Autodesk Fusion 360 part; units mm, degrees
(part 3 of 3)
  spline S35 degree 5 poles (10.6114, 19.2717) (10.6024, 19.2665) (10.5842, 19.256) (10.557, 19.2403) (10.5209, 19.2193) (10.476, 19.1928) (10.4312, 19.1661) (10.3866, 19.1393) (10.3422, 19.1123) (10.298, 19.0851) (10.254, 19.0578) (10.2102, 19.0302) (10.1666, 19.0026) (10.1231, 18.9747) (10.0799, 18.9466) (10.0369, 18.9184) (9.9941, 18.8901) (9.9515, 18.8615) (9.9091, 18.8328) (9.8669, 18.8038) (9.8249, 18.7748) (9.7832, 18.7455) (9.7416, 18.7161) (9.7003, 18.6865) (9.6592, 18.6567) (9.6183, 18.6267) (9.5776, 18.5966) (9.5372, 18.5662) (9.497, 18.5357) (9.457, 18.5051) (9.4173, 18.4742) (9.3778, 18.4432) (9.3385, 18.412) (9.2995, 18.3806) (9.2607, 18.349) (9.2222, 18.3172) (9.1839, 18.2853) (9.1459, 18.2531) (9.1082, 18.2208) (9.0707, 18.1883) (9.0335, 18.1556) (8.9965, 18.1227) (8.9598, 18.0896) (8.9234, 18.0564) (8.8873, 18.0229) (8.8515, 17.9892) (8.816, 17.9554) (8.7808, 17.9213) (8.7458, 17.8871) (8.7112, 17.8526) (8.6769, 17.8179) (8.643, 17.7831) (8.6093, 17.748) (8.576, 17.7127) (8.5431, 17.6772) (8.5105, 17.6415) (8.4782, 17.6055) (8.4464, 17.5693) (8.415, 17.5329) (8.384, 17.4962) (8.3534, 17.4593) (8.3232, 17.4221) (8.2934, 17.3847) (8.264, 17.3471) (8.2352, 17.3092) (8.2069, 17.2709) (8.1792, 17.2323) (8.1523, 17.1934) (8.1261, 17.154) (8.1007, 17.1142) (8.0762, 17.074) (8.0573, 17.0414) (8.0434, 17.0168) (8.0344, 17.0003) (8.0299, 16.992) knots -1 -1 -1 -1 -1 -1 -0.98571429 -0.97142857 -0.95714286 -0.94285714 -0.92857143 -0.91428571 -0.9 -0.88571429 -0.87142857 -0.85714286 -0.84285714 -0.82857143 -0.81428571 -0.8 -0.78571429 -0.77142857 -0.75714286 -0.74285714 -0.72857143 -0.71428571 -0.7 -0.68571429 -0.67142857 -0.65714286 -0.64285714 -0.62857143 -0.61428571 -0.6 -0.58571429 -0.57142857 -0.55714286 -0.54285714 -0.52857143 -0.51428571 -0.5 -0.48571429 -0.47142857 -0.45714286 -0.44285714 -0.42857143 -0.41428571 -0.4 -0.38571429 -0.37142857 -0.35714286 -0.34285714 -0.32857143 -0.31428571 -0.3 -0.28571429 -0.27142857 -0.25714286 -0.24285714 -0.22857143 -0.21428571 -0.2 -0.18571429 -0.17142857 -0.15714286 -0.14285714 -0.12857143 -0.11428571 -0.1 -0.08571429 -0.07142857 -0.05714286 -0.04285714 -0.02857143 -0.01428571 0 0 0 0 0 0
  line L71 (8.0299, 16.992) -> (7.6878, 16.268)
  arc A53 (7.0347, 16.0238) -> (7.6878, 16.268) centre (7.2357, 16.4816) ccw
  arc A54 (7.0347, 16.0238) -> (5.868, 16.4869) centre (0, 0) ccw
  arc A55 (5.5602, 17.1124) -> (5.868, 16.4869) centre (6.0357, 16.9579) ccw
  line L72 (5.5602, 17.1124) -> (5.8076, 17.874)
  spline S36 degree 5 poles (5.8076, 17.874) (5.81, 17.8831) (5.8148, 17.9013) (5.8216, 17.9287) (5.8301, 17.9654) (5.8399, 18.0115) (5.8487, 18.0579) (5.8566, 18.1045) (5.8637, 18.1513) (5.8701, 18.1983) (5.8757, 18.2456) (5.8807, 18.293) (5.8852, 18.3405) (5.8891, 18.3882) (5.8926, 18.4359) (5.8957, 18.4838) (5.8982, 18.5317) (5.9003, 18.5798) (5.902, 18.628) (5.9032, 18.6762) (5.904, 18.7246) (5.9043, 18.773) (5.9043, 18.8216) (5.9039, 18.8702) (5.903, 18.9188) (5.9019, 18.9676) (5.9003, 19.0164) (5.8984, 19.0653) (5.8961, 19.1142) (5.8935, 19.1632) (5.8905, 19.2123) (5.8871, 19.2614) (5.8835, 19.3106) (5.8794, 19.3598) (5.8751, 19.4091) (5.8704, 19.4584) (5.8654, 19.5078) (5.8601, 19.5572) (5.8545, 19.6066) (5.8486, 19.6561) (5.8423, 19.7057) (5.8357, 19.7552) (5.8289, 19.8048) (5.8217, 19.8545) (5.8142, 19.9042) (5.8065, 19.9539) (5.7984, 20.0036) (5.7901, 20.0534) (5.7814, 20.1032) (5.7725, 20.153) (5.7633, 20.2029) (5.7538, 20.2527) (5.744, 20.3026) (5.734, 20.3525) (5.7236, 20.4025) (5.713, 20.4524) (5.7021, 20.5024) (5.691, 20.5524) (5.6796, 20.6024) (5.6679, 20.6524) (5.6559, 20.7024) (5.6437, 20.7525) (5.6312, 20.8026) (5.6184, 20.8526) (5.6054, 20.9027) (5.5921, 20.9528) (5.5786, 21.0029) (5.5648, 21.053) (5.5507, 21.1031) (5.5364, 21.1532) (5.5219, 21.2033) (5.51, 21.2434) (5.501, 21.2734) (5.4949, 21.2935) (5.4919, 21.3035) knots 0 0 0 0 0 0 0.01428571 0.02857143 0.04285714 0.05714286 0.07142857 0.08571429 0.1 0.11428571 0.12857143 0.14285714 0.15714286 0.17142857 0.18571429 0.2 0.21428571 0.22857143 0.24285714 0.25714286 0.27142857 0.28571429 0.3 0.31428571 0.32857143 0.34285714 0.35714286 0.37142857 0.38571429 0.4 0.41428571 0.42857143 0.44285714 0.45714286 0.47142857 0.48571429 0.5 0.51428571 0.52857143 0.54285714 0.55714286 0.57142857 0.58571429 0.6 0.61428571 0.62857143 0.64285714 0.65714286 0.67142857 0.68571429 0.7 0.71428571 0.72857143 0.74285714 0.75714286 0.77142857 0.78571429 0.8 0.81428571 0.82857143 0.84285714 0.85714286 0.87142857 0.88571429 0.9 0.91428571 0.92857143 0.94285714 0.95714286 0.97142857 0.98571429 1 1 1 1 1 1
  line L73 (5.4919, 21.3035) -> (4.8168, 21.4662)
  line L74 (4.8168, 21.4662) -> (4.1368, 21.6076)
  spline S37 degree 5 poles (4.1368, 21.6076) (4.1298, 21.5998) (4.1157, 21.5843) (4.0948, 21.5609) (4.0669, 21.5297) (4.0323, 21.4907) (3.998, 21.4515) (3.9639, 21.4122) (3.93, 21.3728) (3.8964, 21.3333) (3.863, 21.2937) (3.8298, 21.254) (3.7969, 21.2141) (3.7642, 21.1742) (3.7317, 21.1342) (3.6996, 21.0941) (3.6676, 21.0539) (3.6359, 21.0135) (3.6045, 20.9731) (3.5733, 20.9326) (3.5423, 20.8919) (3.5117, 20.8512) (3.4812, 20.8104) (3.4511, 20.7694) (3.4212, 20.7284) (3.3916, 20.6873) (3.3622, 20.646) (3.3331, 20.6047) (3.3043, 20.5633) (3.2758, 20.5217) (3.2475, 20.4801) (3.2195, 20.4384) (3.1918, 20.3966) (3.1644, 20.3546) (3.1373, 20.3126) (3.1105, 20.2705) (3.084, 20.2283) (3.0578, 20.186) (3.0318, 20.1436) (3.0062, 20.1011) (2.9809, 20.0585) (2.956, 20.0158) (2.9313, 19.973) (2.907, 19.9301) (2.883, 19.8871) (2.8593, 19.844) (2.836, 19.8009) (2.813, 19.7576) (2.7904, 19.7142) (2.7681, 19.6708) (2.7462, 19.6272) (2.7247, 19.5835) (2.7035, 19.5398) (2.6828, 19.4959) (2.6624, 19.452) (2.6424, 19.4079) (2.6229, 19.3638) (2.6038, 19.3195) (2.5852, 19.2751) (2.567, 19.2307) (2.5493, 19.1861) (2.5321, 19.1414) (2.5153, 19.0967) (2.499, 19.0518) (2.4833, 19.0068) (2.4682, 18.9617) (2.4538, 18.9164) (2.4402, 18.8711) (2.4275, 18.8255) (2.4157, 18.7798) (2.4048, 18.734) (2.3968, 18.6972) (2.3913, 18.6695) (2.3878, 18.651) (2.3861, 18.6418) knots -1 -1 -1 -1 -1 -1 -0.98571429 -0.97142857 -0.95714286 -0.94285714 -0.92857143 -0.91428571 -0.9 -0.88571429 -0.87142857 -0.85714286 -0.84285714 -0.82857143 -0.81428571 -0.8 -0.78571429 -0.77142857 -0.75714286 -0.74285714 -0.72857143 -0.71428571 -0.7 -0.68571429 -0.67142857 -0.65714286 -0.64285714 -0.62857143 -0.61428571 -0.6 -0.58571429 -0.57142857 -0.55714286 -0.54285714 -0.52857143 -0.51428571 -0.5 -0.48571429 -0.47142857 -0.45714286 -0.44285714 -0.42857143 -0.41428571 -0.4 -0.38571429 -0.37142857 -0.35714286 -0.34285714 -0.32857143 -0.31428571 -0.3 -0.28571429 -0.27142857 -0.25714286 -0.24285714 -0.22857143 -0.21428571 -0.2 -0.18571429 -0.17142857 -0.15714286 -0.14285714 -0.12857143 -0.11428571 -0.1 -0.08571429 -0.07142857 -0.05714286 -0.04285714 -0.02857143 -0.01428571 0 0 0 0 0 0
  line L75 (2.3861, 18.6418) -> (2.2844, 17.8474)
  arc A56 (1.7388, 17.4134) -> (2.2844, 17.8474) centre (1.7885, 17.9109) ccw
  arc A57 (1.7388, 17.4134) -> (0.4861, 17.4932) centre (0, 0) ccw
  arc A58 (0, 17.9931) -> (0.4861, 17.4932) centre (0.5, 17.9931) ccw
  line L76 (0, 17.9931) -> (0, 18.7939)
  spline S38 degree 5 poles (0, 18.7939) (-0.0005, 18.8032) (-0.0016, 18.822) (-0.0036, 18.8502) (-0.0068, 18.8877) (-0.0118, 18.9346) (-0.0178, 18.9814) (-0.0246, 19.0282) (-0.0323, 19.0749) (-0.0408, 19.1216) (-0.0501, 19.1683) (-0.06, 19.2149) (-0.0704, 19.2615) (-0.0814, 19.308) (-0.0928, 19.3545) (-0.1047, 19.401) (-0.1171, 19.4474) (-0.1299, 19.4937) (-0.1432, 19.5401) (-0.157, 19.5863) (-0.1712, 19.6326) (-0.1858, 19.6788) (-0.2009, 19.7249) (-0.2163, 19.771) (-0.2321, 19.817) (-0.2483, 19.863) (-0.2649, 19.909) (-0.2818, 19.9549) (-0.2991, 20.0007) (-0.3167, 20.0465) (-0.3347, 20.0922) (-0.3531, 20.1379) (-0.3718, 20.1835) (-0.3908, 20.2291) (-0.4102, 20.2746) (-0.4299, 20.3201) (-0.4499, 20.3655) (-0.4702, 20.4109) (-0.4908, 20.4561) (-0.5118, 20.5014) (-0.533, 20.5466) (-0.5546, 20.5917) (-0.5764, 20.6367) (-0.5986, 20.6817) (-0.6211, 20.7267) (-0.6438, 20.7716) (-0.6668, 20.8164) (-0.6902, 20.8611) (-0.7138, 20.9058) (-0.7376, 20.9504) (-0.7618, 20.995) (-0.7863, 21.0395) (-0.811, 21.0839) (-0.836, 21.1283) (-0.8612, 21.1726) (-0.8867, 21.2168) (-0.9125, 21.261) (-0.9386, 21.3051) (-0.9649, 21.3491) (-0.9915, 21.3931) (-1.0183, 21.437) (-1.0454, 21.4808) (-1.0728, 21.5245) (-1.1004, 21.5682) (-1.1282, 21.6118) (-1.1563, 21.6553) (-1.1847, 21.6988) (-1.2133, 21.7422) (-1.2421, 21.7855) (-1.2712, 21.8287) (-1.3006, 21.8719) (-1.3242, 21.9063) (-1.3421, 21.9321) (-1.354, 21.9493) (-1.36, 21.9579) knots 0 0 0 0 0 0 0.01428571 0.02857143 0.04285714 0.05714286 0.07142857 0.08571429 0.1 0.11428571 0.12857143 0.14285714 0.15714286 0.17142857 0.18571429 0.2 0.21428571 0.22857143 0.24285714 0.25714286 0.27142857 0.28571429 0.3 0.31428571 0.32857143 0.34285714 0.35714286 0.37142857 0.38571429 0.4 0.41428571 0.42857143 0.44285714 0.45714286 0.47142857 0.48571429 0.5 0.51428571 0.52857143 0.54285714 0.55714286 0.57142857 0.58571429 0.6 0.61428571 0.62857143 0.64285714 0.65714286 0.67142857 0.68571429 0.7 0.71428571 0.72857143 0.74285714 0.75714286 0.77142857 0.78571429 0.8 0.81428571 0.82857143 0.84285714 0.85714286 0.87142857 0.88571429 0.9 0.91428571 0.92857143 0.94285714 0.95714286 0.97142857 0.98571429 1 1 1 1 1 1
  line L77 (-1.36, 21.9579) -> (-2.0524, 21.9041)
  line L78 (-2.0524, 21.9041) -> (-2.7428, 21.8284)
  spline S39 degree 5 poles (-2.7428, 21.8284) (-2.747, 21.8188) (-2.7556, 21.7997) (-2.7683, 21.771) (-2.7852, 21.7327) (-2.806, 21.6849) (-2.8265, 21.637) (-2.8468, 21.5891) (-2.8669, 21.5412) (-2.8867, 21.4932) (-2.9062, 21.4452) (-2.9255, 21.3972) (-2.9445, 21.3491) (-2.9632, 21.3011) (-2.9817, 21.253) (-2.9999, 21.2049) (-3.0179, 21.1568) (-3.0356, 21.1086) (-3.053, 21.0604) (-3.0701, 21.0123) (-3.087, 20.964) (-3.1036, 20.9158) (-3.1199, 20.8676) (-3.1359, 20.8193) (-3.1517, 20.7711) (-3.1672, 20.7228) (-3.1823, 20.6745) (-3.1972, 20.6262) (-3.2118, 20.5779) (-3.2261, 20.5296) (-3.2401, 20.4813) (-3.2539, 20.4329) (-3.2673, 20.3846) (-3.2804, 20.3363) (-3.2932, 20.2879) (-3.3057, 20.2396) (-3.3179, 20.1913) (-3.3297, 20.1429) (-3.3413, 20.0946) (-3.3525, 20.0462) (-3.3634, 19.9979) (-3.3739, 19.9496) (-3.3842, 19.9013) (-3.3941, 19.853) (-3.4036, 19.8047) (-3.4128, 19.7564) (-3.4216, 19.7081) (-3.4301, 19.6599) (-3.4382, 19.6116) (-3.446, 19.5634) (-3.4533, 19.5152) (-3.4603, 19.467) (-3.4669, 19.4189) (-3.4731, 19.3707) (-3.4789, 19.3226) (-3.4843, 19.2746) (-3.4892, 19.2265) (-3.4937, 19.1786) (-3.4977, 19.1306) (-3.5012, 19.0827) (-3.5043, 19.0349) (-3.5069, 18.987) (-3.509, 18.9393) (-3.5106, 18.8916) (-3.5117, 18.8439) (-3.5121, 18.7963) (-3.5118, 18.7489) (-3.5107, 18.7015) (-3.5087, 18.6543) (-3.5058, 18.6072) (-3.502, 18.5602) (-3.4982, 18.5227) (-3.4949, 18.4947) (-3.4926, 18.476) (-3.4913, 18.4667) knots -1 -1 -1 -1 -1 -1 -0.98571429 -0.97142857 -0.95714286 -0.94285714 -0.92857143 -0.91428571 -0.9 -0.88571429 -0.87142857 -0.85714286 -0.84285714 -0.82857143 -0.81428571 -0.8 -0.78571429 -0.77142857 -0.75714286 -0.74285714 -0.72857143 -0.71428571 -0.7 -0.68571429 -0.67142857 -0.65714286 -0.64285714 -0.62857143 -0.61428571 -0.6 -0.58571429 -0.57142857 -0.55714286 -0.54285714 -0.52857143 -0.51428571 -0.5 -0.48571429 -0.47142857 -0.45714286 -0.44285714 -0.42857143 -0.41428571 -0.4 -0.38571429 -0.37142857 -0.35714286 -0.34285714 -0.32857143 -0.31428571 -0.3 -0.28571429 -0.27142857 -0.25714286 -0.24285714 -0.22857143 -0.21428571 -0.2 -0.18571429 -0.17142857 -0.15714286 -0.14285714 -0.12857143 -0.11428571 -0.1 -0.08571429 -0.07142857 -0.05714286 -0.04285714 -0.02857143 -0.01428571 0 0 0 0 0 0
  line L79 (-3.4913, 18.4667) -> (-3.3426, 17.6799)
  arc A59 (-3.7274, 17.0984) -> (-3.3426, 17.6799) centre (-3.8339, 17.587) ccw
  arc A60 (-3.7274, 17.0984) -> (-4.9434, 16.7873) centre (0, 0) ccw
  arc A61 (-17.151, -5.4413) -> (-16.9072, -4.9787) centre (-17.2669, -5.0846) ccw
  arc A62 (-17.2206, -3.754) -> (-16.9072, -4.9787) centre (0, 0) ccw
  arc A63 (-17.2206, -3.754) -> (-17.6566, -3.4654) centre (-17.587, -3.8339) ccw
  line L80 (-18.4469, -3.6148) -> (-17.6566, -3.4654)
  spline S40 degree 3 poles (-21.9448, -2.8275) (-21.9231, -2.8373) (-21.9013, -2.847) (-21.8795, -2.8568) (-21.1038, -3.2048) (-20.3139, -3.4618) (-19.5249, -3.5782) (-19.1675, -3.6309) (-18.8078, -3.6627) (-18.4503, -3.6152) (-18.4491, -3.6151) (-18.448, -3.6149) (-18.4469, -3.6148) knots -1.019521 -1.019521 -1.019521 -1.019521 -1 -1 -1 -0.311758 -0.311758 -0.311758 0 0 0 0.001043 0.001043 0.001043 0.001043
  line L81 (-22.0285, -2.0641) -> (-21.9448, -2.8275)
  line L82 (-22.0881, -1.2984) -> (-22.0285, -2.0641)
  spline S41 degree 3 poles (-18.7973, 0.125) (-18.7984, 0.1249) (-18.7996, 0.1249) (-18.8007, 0.1248) (-19.3678, 0.0936) (-19.9052, -0.1072) (-20.433, -0.3432) (-20.9804, -0.5879) (-21.5134, -0.8979) (-22.0294, -1.2575) (-22.049, -1.2711) (-22.0685, -1.2847) (-22.0881, -1.2984) knots -0.001043 -0.001043 -0.001043 -0.001043 0 0 0 0.490911 0.490911 0.490911 1 1 1 1.019521 1.019521 1.019521 1.019521
  line L83 (-17.9931, 0.125) -> (-18.7973, 0.125)
  arc A64 (-17.9931, 0.125) -> (-17.6182, 0.4896) centre (-17.9931, 0.5) ccw
  arc A65 (-17.5378, 1.7512) -> (-17.6182, 0.4896) centre (0, 0) ccw
  arc A66 (-17.5378, 1.7512) -> (-17.8633, 2.1604) centre (-17.9109, 1.7885) ccw
  line L84 (-18.661, 2.2625) -> (-17.8633, 2.1604)
  spline S42 degree 3 poles (-21.7445, 4.0922) (-21.7268, 4.0762) (-21.7091, 4.0602) (-21.6915, 4.0442) (-21.0612, 3.4735) (-20.3894, 2.985) (-19.675, 2.6305) (-19.3514, 2.4699) (-19.0191, 2.3285) (-18.6644, 2.2632) (-18.6633, 2.2629) (-18.6622, 2.2627) (-18.661, 2.2625) knots -1.019521 -1.019521 -1.019521 -1.019521 -1 -1 -1 -0.311758 -0.311758 -0.311758 0 0 0 0.001043 0.001043 0.001043 0.001043
  line L85 (-21.5882, 4.8441) -> (-21.7445, 4.0922)
  line L86 (-21.4082, 5.5908) -> (-21.5882, 4.8441)
  spline S43 degree 3 poles (-17.8387, 5.9276) (-17.8398, 5.9279) (-17.8409, 5.9281) (-17.842, 5.9284) (-18.391, 6.074) (-18.9641, 6.0491) (-19.539, 5.9878) (-20.1352, 5.9242) (-20.7379, 5.794) (-21.3398, 5.6115) (-21.3626, 5.6046) (-21.3854, 5.5977) (-21.4082, 5.5908) knots -0.001043 -0.001043 -0.001043 -0.001043 0 0 0 0.490911 0.490911 0.490911 1 1 1 1.019521 1.019521 1.019521 1.019521
  line L87 (-17.0738, 5.679) -> (-17.8387, 5.9276)
  arc A67 (-17.0738, 5.679) -> (-16.6046, 5.9099) centre (-16.9579, 6.0357) ccw
  arc A68 (-16.1383, 7.085) -> (-16.6046, 5.9099) centre (0, 0) ccw
  arc A69 (-16.1383, 7.085) -> (-16.3214, 7.5748) centre (-16.4816, 7.2357) ccw
  line L88 (-17.0485, 7.9184) -> (-16.3214, 7.5748)
  spline S44 degree 3 poles (-19.4157, 10.6113) (-19.4038, 10.5906) (-19.392, 10.5699) (-19.3801, 10.5493) (-18.9571, 9.8117) (-18.4691, 9.1396) (-17.8992, 8.5817) (-17.641, 8.329) (-17.3687, 8.0918) (-17.0516, 7.92) (-17.0506, 7.9195) (-17.0496, 7.9189) (-17.0485, 7.9184) knots -1.019521 -1.019521 -1.019521 -1.019521 -1 -1 -1 -0.311758 -0.311758 -0.311758 0 0 0 0.001043 0.001043 0.001043 0.001043
  line L89 (-19.0347, 11.2782) -> (-19.4157, 10.6113)
  line L90 (-18.6328, 11.9326) -> (-19.0347, 11.2782)
  spline S45 degree 3 poles (-15.1339, 11.1499) (-15.1348, 11.1505) (-15.1358, 11.1511) (-15.1367, 11.1518) (-15.6139, 11.4599) (-16.1667, 11.6132) (-16.7324, 11.7326) (-17.319, 11.8564) (-17.9325, 11.9188) (-18.5613, 11.9312) (-18.5851, 11.9317) (-18.609, 11.9322) (-18.6328, 11.9326) knots -0.001043 -0.001043 -0.001043 -0.001043 0 0 0 0.490911 0.490911 0.490911 1 1 1 1.019521 1.019521 1.019521 1.019521
  line L91 (-14.4832, 10.6772) -> (-15.1339, 11.1499)
  arc A70 (-14.4832, 10.6772) -> (-13.9657, 10.7518) centre (-14.2628, 10.9806) ccw
  arc A71 (-13.159, 11.7252) -> (-13.9657, 10.7518) centre (0, 0) ccw
  arc A72 (-13.159, 11.7252) -> (-13.1819, 12.2476) centre (-13.439, 11.9747) ccw
  line L92 (-13.7672, 12.7991) -> (-13.1819, 12.2476)
  spline S46 degree 3 poles (-15.1864, 16.0918) (-15.1815, 16.0684) (-15.1766, 16.0451) (-15.1717, 16.0217) (-14.9972, 15.1896) (-14.7409, 14.3995) (-14.3712, 13.6928) (-14.2038, 13.3727) (-14.0181, 13.063) (-13.7696, 12.8016) (-13.7688, 12.8008) (-13.768, 12.7999) (-13.7672, 12.7991) knots -1.019521 -1.019521 -1.019521 -1.019521 -1 -1 -1 -0.311758 -0.311758 -0.311758 0 0 0 0.001043 0.001043 0.001043 0.001043
  line L93 (-14.6179, 16.6082) -> (-15.1864, 16.0918)
  line L94 (-14.0335, 17.1065) -> (-14.6179, 16.6082)
  spline S47 degree 3 poles (-10.9476, 15.2808) (-10.9484, 15.2817) (-10.9491, 15.2826) (-10.9498, 15.2835) (-11.3084, 15.7239) (-11.7867, 16.0406) (-12.2879, 16.3289) (-12.8075, 16.6279) (-13.3717, 16.8769) (-13.9659, 17.083) (-13.9884, 17.0908) (-14.0109, 17.0987) (-14.0335, 17.1065) knots -0.001043 -0.001043 -0.001043 -0.001043 0 0 0 0.490911 0.490911 0.490911 1 1 1 1.019521 1.019521 1.019521 1.019521
  line L95 (-10.4749, 14.6302) -> (-10.9476, 15.2808)
  arc A73 (-10.4749, 14.6302) -> (-9.9596, 14.5412) centre (-10.1715, 14.8506) ccw
  arc A74 (-8.8917, 15.2177) -> (-9.9596, 14.5412) centre (0, 0) ccw
  arc A75 (-8.8917, 15.2177) -> (-8.752, 15.7216) centre (-9.0809, 15.5415) ccw
  line L96 (-9.1383, 16.427) -> (-8.752, 15.7216)
  spline S48 degree 3 poles (-9.4705, 19.997) (-9.473, 19.9733) (-9.4756, 19.9496) (-9.4781, 19.9259) (-9.5694, 19.0805) (-9.5697, 18.2499) (-9.4366, 17.4636) (-9.3763, 17.1074) (-9.2954, 16.7555) (-9.1397, 16.4301) (-9.1392, 16.429) (-9.1388, 16.428) (-9.1383, 16.427) knots -1.019521 -1.019521 -1.019521 -1.019521 -1 -1 -1 -0.311758 -0.311758 -0.311758 0 0 0 0.001043 0.001043 0.001043 0.001043
  line L97 (-8.7702, 20.3125) -> (-9.4705, 19.997)
  line L98 (-8.0604, 20.6058) -> (-8.7702, 20.3125)
  spline S49 degree 3 poles (-5.6898, 17.9159) (-5.6902, 17.917) (-5.6906, 17.918) (-5.691, 17.9191) (-5.8959, 18.4488) (-6.253, 18.8978) (-6.6405, 19.3269) (-7.0424, 19.7718) (-7.502, 20.183) (-8.0034, 20.5626) (-8.0224, 20.577) (-8.0414, 20.5914) (-8.0604, 20.6058) knots -0.001043 -0.001043 -0.001043 -0.001043 0 0 0 0.490911 0.490911 0.490911 1 1 1 1.019521 1.019521 1.019521 1.019521
  line L99 (-5.4413, 17.151) -> (-5.6898, 17.9159)
  arc A76 (-5.4413, 17.151) -> (-4.9787, 16.9072) centre (-5.0846, 17.2669) ccw
  arc A77 (-3.754, 17.2206) -> (-4.9787, 16.9072) centre (0, 0) ccw
  arc A78 (-3.754, 17.2206) -> (-3.4654, 17.6566) centre (-3.8339, 17.587) ccw
  line L100 (-3.6148, 18.4469) -> (-3.4654, 17.6566)
  spline S50 degree 3 poles (-2.8275, 21.9448) (-2.8373, 21.9231) (-2.847, 21.9013) (-2.8568, 21.8795) (-3.2048, 21.1038) (-3.4618, 20.3139) (-3.5782, 19.5249) (-3.6309, 19.1675) (-3.6627, 18.8078) (-3.6152, 18.4503) (-3.6151, 18.4491) (-3.6149, 18.448) (-3.6148, 18.4469) knots -1.019521 -1.019521 -1.019521 -1.019521 -1 -1 -1 -0.311758 -0.311758 -0.311758 0 0 0 0.001043 0.001043 0.001043 0.001043
  line L101 (-2.0641, 22.0285) -> (-2.8275, 21.9448)
  line L102 (-1.2984, 22.0881) -> (-2.0641, 22.0285)
  spline S51 degree 3 poles (0.125, 18.7973) (0.1249, 18.7984) (0.1249, 18.7996) (0.1248, 18.8007) (0.0936, 19.3678) (-0.1072, 19.9052) (-0.3432, 20.433) (-0.5879, 20.9804) (-0.8979, 21.5134) (-1.2575, 22.0294) (-1.2711, 22.049) (-1.2847, 22.0685) (-1.2984, 22.0881) knots -0.001043 -0.001043 -0.001043 -0.001043 0 0 0 0.490911 0.490911 0.490911 1 1 1 1.019521 1.019521 1.019521 1.019521
  line L103 (0.125, 17.9931) -> (0.125, 18.7973)
  arc A79 (0.125, 17.9931) -> (0.4896, 17.6182) centre (0.5, 17.9931) ccw
  arc A80 (1.7512, 17.5378) -> (0.4896, 17.6182) centre (0, 0) ccw
  arc A81 (1.7512, 17.5378) -> (2.1604, 17.8633) centre (1.7885, 17.9109) ccw
  line L104 (2.2625, 18.661) -> (2.1604, 17.8633)
  spline S52 degree 3 poles (4.0922, 21.7445) (4.0762, 21.7268) (4.0602, 21.7091) (4.0442, 21.6915) (3.4735, 21.0612) (2.985, 20.3894) (2.6305, 19.675) (2.4699, 19.3514) (2.3285, 19.0191) (2.2632, 18.6644) (2.2629, 18.6633) (2.2627, 18.6622) (2.2625, 18.661) knots -1.019521 -1.019521 -1.019521 -1.019521 -1 -1 -1 -0.311758 -0.311758 -0.311758 0 0 0 0.001043 0.001043 0.001043 0.001043
  line L105 (4.8441, 21.5882) -> (4.0922, 21.7445)
  line L106 (5.5908, 21.4082) -> (4.8441, 21.5882)
  spline S53 degree 3 poles (5.9276, 17.8387) (5.9279, 17.8398) (5.9281, 17.8409) (5.9284, 17.842) (6.074, 18.391) (6.0491, 18.9641) (5.9878, 19.539) (5.9242, 20.1352) (5.794, 20.7379) (5.6115, 21.3398) (5.6046, 21.3626) (5.5977, 21.3854) (5.5908, 21.4082) knots -0.001043 -0.001043 -0.001043 -0.001043 0 0 0 0.490911 0.490911 0.490911 1 1 1 1.019521 1.019521 1.019521 1.019521
  line L107 (5.679, 17.0738) -> (5.9276, 17.8387)
  arc A82 (5.679, 17.0738) -> (5.9099, 16.6046) centre (6.0357, 16.9579) ccw
  arc A83 (7.085, 16.1383) -> (5.9099, 16.6046) centre (0, 0) ccw
  arc A84 (7.085, 16.1383) -> (7.5748, 16.3214) centre (7.2357, 16.4816) ccw
  line L108 (7.9184, 17.0485) -> (7.5748, 16.3214)
  spline S54 degree 3 poles (10.6113, 19.4157) (10.5906, 19.4038) (10.5699, 19.392) (10.5493, 19.3801) (9.8117, 18.9571) (9.1396, 18.4691) (8.5817, 17.8992) (8.329, 17.641) (8.0918, 17.3687) (7.92, 17.0516) (7.9195, 17.0506) (7.9189, 17.0496) (7.9184, 17.0485) knots -1.019521 -1.019521 -1.019521 -1.019521 -1 -1 -1 -0.311758 -0.311758 -0.311758 0 0 0 0.001043 0.001043 0.001043 0.001043
  line L109 (11.2782, 19.0347) -> (10.6113, 19.4157)
  line L110 (11.9326, 18.6328) -> (11.2782, 19.0347)
  spline S55 degree 3 poles (11.1499, 15.1339) (11.1505, 15.1348) (11.1511, 15.1358) (11.1518, 15.1367) (11.4599, 15.6139) (11.6132, 16.1667) (11.7326, 16.7324) (11.8564, 17.319) (11.9188, 17.9325) (11.9312, 18.5613) (11.9317, 18.5851) (11.9322, 18.609) (11.9326, 18.6328) knots -0.001043 -0.001043 -0.001043 -0.001043 0 0 0 0.490911 0.490911 0.490911 1 1 1 1.019521 1.019521 1.019521 1.019521
  line L111 (10.6772, 14.4832) -> (11.1499, 15.1339)
  arc A85 (10.6772, 14.4832) -> (10.7518, 13.9657) centre (10.9806, 14.2628) ccw
  arc A86 (11.7252, 13.159) -> (10.7518, 13.9657) centre (0, 0) ccw
  arc A87 (11.7252, 13.159) -> (12.2476, 13.1819) centre (11.9747, 13.439) ccw
  line L112 (12.7991, 13.7672) -> (12.2476, 13.1819)
  spline S56 degree 3 poles (16.0918, 15.1864) (16.0684, 15.1815) (16.0451, 15.1766) (16.0217, 15.1717) (15.1896, 14.9972) (14.3995, 14.7409) (13.6928, 14.3712) (13.3727, 14.2038) (13.063, 14.0181) (12.8016, 13.7696) (12.8008, 13.7688) (12.7999, 13.768) (12.7991, 13.7672) knots -1.019521 -1.019521 -1.019521 -1.019521 -1 -1 -1 -0.311758 -0.311758 -0.311758 0 0 0 0.001043 0.001043 0.001043 0.001043
  line L113 (16.6082, 14.6179) -> (16.0918, 15.1864)
  line L114 (17.1065, 14.0335) -> (16.6082, 14.6179)
  spline S57 degree 3 poles (15.2808, 10.9476) (15.2817, 10.9484) (15.2826, 10.9491) (15.2835, 10.9498) (15.7239, 11.3084) (16.0406, 11.7867) (16.3289, 12.2879) (16.6279, 12.8075) (16.8769, 13.3717) (17.083, 13.9659) (17.0908, 13.9884) (17.0987, 14.0109) (17.1065, 14.0335) knots -0.001043 -0.001043 -0.001043 -0.001043 0 0 0 0.490911 0.490911 0.490911 1 1 1 1.019521 1.019521 1.019521 1.019521
  line L115 (14.6302, 10.4749) -> (15.2808, 10.9476)
  arc A88 (14.6302, 10.4749) -> (14.5412, 9.9596) centre (14.8506, 10.1715) ccw
  arc A89 (15.2177, 8.8917) -> (14.5412, 9.9596) centre (0, 0) ccw
  arc A90 (15.2177, 8.8917) -> (15.7216, 8.752) centre (15.5415, 9.0809) ccw
  line L116 (16.427, 9.1383) -> (15.7216, 8.752)
  spline S58 degree 3 poles (19.997, 9.4705) (19.9733, 9.473) (19.9496, 9.4756) (19.9259, 9.4781) (19.0805, 9.5694) (18.2499, 9.5697) (17.4636, 9.4366) (17.1074, 9.3763) (16.7555, 9.2954) (16.4301, 9.1397) (16.429, 9.1392) (16.428, 9.1388) (16.427, 9.1383) knots -1.019521 -1.019521 -1.019521 -1.019521 -1 -1 -1 -0.311758 -0.311758 -0.311758 0 0 0 0.001043 0.001043 0.001043 0.001043
  line L117 (20.3125, 8.7702) -> (19.997, 9.4705)
  line L118 (20.6058, 8.0604) -> (20.3125, 8.7702)
  spline S59 degree 3 poles (17.9159, 5.6898) (17.917, 5.6902) (17.918, 5.6906) (17.9191, 5.691) (18.4488, 5.8959) (18.8978, 6.253) (19.3269, 6.6405) (19.7718, 7.0424) (20.183, 7.502) (20.5626, 8.0034) (20.577, 8.0224) (20.5914, 8.0414) (20.6058, 8.0604) knots -0.001043 -0.001043 -0.001043 -0.001043 0 0 0 0.490911 0.490911 0.490911 1 1 1 1.019521 1.019521 1.019521 1.019521
  line L119 (17.151, 5.4413) -> (17.9159, 5.6898)
  arc A91 (17.151, 5.4413) -> (16.9072, 4.9787) centre (17.2669, 5.0846) ccw
  arc A92 (17.2206, 3.754) -> (16.9072, 4.9787) centre (0, 0) ccw
  arc A93 (17.2206, 3.754) -> (17.6566, 3.4654) centre (17.587, 3.8339) ccw
  line L120 (18.4469, 3.6148) -> (17.6566, 3.4654)
  spline S60 degree 3 poles (21.9448, 2.8275) (21.9231, 2.8373) (21.9013, 2.847) (21.8795, 2.8568) (21.1038, 3.2048) (20.3139, 3.4618) (19.5249, 3.5782) (19.1675, 3.6309) (18.8078, 3.6627) (18.4503, 3.6152) (18.4491, 3.6151) (18.448, 3.6149) (18.4469, 3.6148) knots -1.019521 -1.019521 -1.019521 -1.019521 -1 -1 -1 -0.311758 -0.311758 -0.311758 0 0 0 0.001043 0.001043 0.001043 0.001043
  line L121 (22.0285, 2.0641) -> (21.9448, 2.8275)
  line L122 (22.0881, 1.2984) -> (22.0285, 2.0641)
  spline S61 degree 3 poles (18.7973, -0.125) (18.7984, -0.1249) (18.7996, -0.1249) (18.8007, -0.1248) (19.3678, -0.0936) (19.9052, 0.1072) (20.433, 0.3432) (20.9804, 0.5879) (21.5134, 0.8979) (22.0294, 1.2575) (22.049, 1.2711) (22.0685, 1.2847) (22.0881, 1.2984) knots -0.001043 -0.001043 -0.001043 -0.001043 0 0 0 0.490911 0.490911 0.490911 1 1 1 1.019521 1.019521 1.019521 1.019521
  line L123 (17.9931, -0.125) -> (18.7973, -0.125)
  arc A94 (17.9931, -0.125) -> (17.6182, -0.4896) centre (17.9931, -0.5) ccw
  arc A95 (17.5378, -1.7512) -> (17.6182, -0.4896) centre (0, 0) ccw
  arc A96 (17.5378, -1.7512) -> (17.8633, -2.1604) centre (17.9109, -1.7885) ccw
  line L124 (18.661, -2.2625) -> (17.8633, -2.1604)
  spline S62 degree 3 poles (21.7445, -4.0922) (21.7268, -4.0762) (21.7091, -4.0602) (21.6915, -4.0442) (21.0612, -3.4735) (20.3894, -2.985) (19.675, -2.6305) (19.3514, -2.4699) (19.0191, -2.3285) (18.6644, -2.2632) (18.6633, -2.2629) (18.6622, -2.2627) (18.661, -2.2625) knots -1.019521 -1.019521 -1.019521 -1.019521 -1 -1 -1 -0.311758 -0.311758 -0.311758 0 0 0 0.001043 0.001043 0.001043 0.001043
  line L125 (21.5882, -4.8441) -> (21.7445, -4.0922)
  line L126 (21.4082, -5.5908) -> (21.5882, -4.8441)
  spline S63 degree 3 poles (17.8387, -5.9276) (17.8398, -5.9279) (17.8409, -5.9281) (17.842, -5.9284) (18.391, -6.074) (18.9641, -6.0491) (19.539, -5.9878) (20.1352, -5.9242) (20.7379, -5.794) (21.3398, -5.6115) (21.3626, -5.6046) (21.3854, -5.5977) (21.4082, -5.5908) knots -0.001043 -0.001043 -0.001043 -0.001043 0 0 0 0.490911 0.490911 0.490911 1 1 1 1.019521 1.019521 1.019521 1.019521
  line L127 (17.0738, -5.679) -> (17.8387, -5.9276)
  arc A97 (17.0738, -5.679) -> (16.6046, -5.9099) centre (16.9579, -6.0357) ccw
  arc A98 (16.1383, -7.085) -> (16.6046, -5.9099) centre (0, 0) ccw
  arc A99 (16.1383, -7.085) -> (16.3214, -7.5748) centre (16.4816, -7.2357) ccw
  line L128 (17.0485, -7.9184) -> (16.3214, -7.5748)
  spline S64 degree 3 poles (19.4157, -10.6113) (19.4038, -10.5906) (19.392, -10.5699) (19.3801, -10.5493) (18.9571, -9.8117) (18.4691, -9.1396) (17.8992, -8.5817) (17.641, -8.329) (17.3687, -8.0918) (17.0516, -7.92) (17.0506, -7.9195) (17.0496, -7.9189) (17.0485, -7.9184) knots -1.019521 -1.019521 -1.019521 -1.019521 -1 -1 -1 -0.311758 -0.311758 -0.311758 0 0 0 0.001043 0.001043 0.001043 0.001043
  line L129 (19.0347, -11.2782) -> (19.4157, -10.6113)
  line L130 (18.6328, -11.9326) -> (19.0347, -11.2782)
  spline S65 degree 3 poles (15.1339, -11.1499) (15.1348, -11.1505) (15.1358, -11.1511) (15.1367, -11.1518) (15.6139, -11.4599) (16.1667, -11.6132) (16.7324, -11.7326) (17.319, -11.8564) (17.9325, -11.9188) (18.5613, -11.9312) (18.5851, -11.9317) (18.609, -11.9322) (18.6328, -11.9326) knots -0.001043 -0.001043 -0.001043 -0.001043 0 0 0 0.490911 0.490911 0.490911 1 1 1 1.019521 1.019521 1.019521 1.019521
  line L131 (14.4832, -10.6772) -> (15.1339, -11.1499)
  arc A100 (14.4832, -10.6772) -> (13.9657, -10.7518) centre (14.2628, -10.9806) ccw
  arc A101 (13.159, -11.7252) -> (13.9657, -10.7518) centre (0, 0) ccw
  arc A102 (13.159, -11.7252) -> (13.1819, -12.2476) centre (13.439, -11.9747) ccw
  line L132 (13.7672, -12.7991) -> (13.1819, -12.2476)
  spline S66 degree 3 poles (15.1864, -16.0918) (15.1815, -16.0684) (15.1766, -16.0451) (15.1717, -16.0217) (14.9972, -15.1896) (14.7409, -14.3995) (14.3712, -13.6928) (14.2038, -13.3727) (14.0181, -13.063) (13.7696, -12.8016) (13.7688, -12.8008) (13.768, -12.7999) (13.7672, -12.7991) knots -1.019521 -1.019521 -1.019521 -1.019521 -1 -1 -1 -0.311758 -0.311758 -0.311758 0 0 0 0.001043 0.001043 0.001043 0.001043
  line L133 (14.6179, -16.6082) -> (15.1864, -16.0918)
  line L134 (14.0335, -17.1065) -> (14.6179, -16.6082)
  spline S67 degree 3 poles (10.9476, -15.2808) (10.9484, -15.2817) (10.9491, -15.2826) (10.9498, -15.2835) (11.3084, -15.7239) (11.7867, -16.0406) (12.2879, -16.3289) (12.8075, -16.6279) (13.3717, -16.8769) (13.9659, -17.083) (13.9884, -17.0908) (14.0109, -17.0987) (14.0335, -17.1065) knots -0.001043 -0.001043 -0.001043 -0.001043 0 0 0 0.490911 0.490911 0.490911 1 1 1 1.019521 1.019521 1.019521 1.019521
  line L135 (10.4749, -14.6302) -> (10.9476, -15.2808)
  arc A103 (10.4749, -14.6302) -> (9.9596, -14.5412) centre (10.1715, -14.8506) ccw
  arc A104 (8.8917, -15.2177) -> (9.9596, -14.5412) centre (0, 0) ccw
  arc A105 (8.8917, -15.2177) -> (8.752, -15.7216) centre (9.0809, -15.5415) ccw
  line L136 (9.1383, -16.427) -> (8.752, -15.7216)
  spline S68 degree 3 poles (9.4705, -19.997) (9.473, -19.9733) (9.4756, -19.9496) (9.4781, -19.9259) (9.5694, -19.0805) (9.5697, -18.2499) (9.4366, -17.4636) (9.3763, -17.1074) (9.2954, -16.7555) (9.1397, -16.4301) (9.1392, -16.429) (9.1388, -16.428) (9.1383, -16.427) knots -1.019521 -1.019521 -1.019521 -1.019521 -1 -1 -1 -0.311758 -0.311758 -0.311758 0 0 0 0.001043 0.001043 0.001043 0.001043
  line L137 (8.7702, -20.3125) -> (9.4705, -19.997)
  line L138 (8.0604, -20.6058) -> (8.7702, -20.3125)
  spline S69 degree 3 poles (5.6898, -17.9159) (5.6902, -17.917) (5.6906, -17.918) (5.691, -17.9191) (5.8959, -18.4488) (6.253, -18.8978) (6.6405, -19.3269) (7.0424, -19.7718) (7.502, -20.183) (8.0034, -20.5626) (8.0224, -20.577) (8.0414, -20.5914) (8.0604, -20.6058) knots -0.001043 -0.001043 -0.001043 -0.001043 0 0 0 0.490911 0.490911 0.490911 1 1 1 1.019521 1.019521 1.019521 1.019521
  line L139 (5.4413, -17.151) -> (5.6898, -17.9159)
  arc A106 (5.4413, -17.151) -> (4.9787, -16.9072) centre (5.0846, -17.2669) ccw
  arc A107 (3.754, -17.2206) -> (4.9787, -16.9072) centre (0, 0) ccw
  arc A108 (3.754, -17.2206) -> (3.4654, -17.6566) centre (3.8339, -17.587) ccw
  line L140 (3.6148, -18.4469) -> (3.4654, -17.6566)
  spline S70 degree 3 poles (2.8275, -21.9448) (2.8373, -21.9231) (2.847, -21.9013) (2.8568, -21.8795) (3.2048, -21.1038) (3.4618, -20.3139) (3.5782, -19.5249) (3.6309, -19.1675) (3.6627, -18.8078) (3.6152, -18.4503) (3.6151, -18.4491) (3.6149, -18.448) (3.6148, -18.4469) knots -1.019521 -1.019521 -1.019521 -1.019521 -1 -1 -1 -0.311758 -0.311758 -0.311758 0 0 0 0.001043 0.001043 0.001043 0.001043
  line L141 (2.0641, -22.0285) -> (2.8275, -21.9448)
  line L142 (1.2984, -22.0881) -> (2.0641, -22.0285)
  spline S71 degree 3 poles (-0.125, -18.7973) (-0.1249, -18.7984) (-0.1249, -18.7996) (-0.1248, -18.8007) (-0.0936, -19.3678) (0.1072, -19.9052) (0.3432, -20.433) (0.5879, -20.9804) (0.8979, -21.5134) (1.2575, -22.0294) (1.2711, -22.049) (1.2847, -22.0685) (1.2984, -22.0881) knots -0.001043 -0.001043 -0.001043 -0.001043 0 0 0 0.490911 0.490911 0.490911 1 1 1 1.019521 1.019521 1.019521 1.019521
  line L143 (-0.125, -17.9931) -> (-0.125, -18.7973)
  arc A109 (-0.125, -17.9931) -> (-0.4896, -17.6182) centre (-0.5, -17.9931) ccw
  arc A110 (-1.7512, -17.5378) -> (-0.4896, -17.6182) centre (0, 0) ccw
  arc A111 (-1.7512, -17.5378) -> (-2.1604, -17.8633) centre (-1.7885, -17.9109) ccw
  line L144 (-2.2625, -18.661) -> (-2.1604, -17.8633)
  spline S72 degree 3 poles (-4.0922, -21.7445) (-4.0762, -21.7268) (-4.0602, -21.7091) (-4.0442, -21.6915) (-3.4735, -21.0612) (-2.985, -20.3894) (-2.6305, -19.675) (-2.4699, -19.3514) (-2.3285, -19.0191) (-2.2632, -18.6644) (-2.2629, -18.6633) (-2.2627, -18.6622) (-2.2625, -18.661) knots -1.019521 -1.019521 -1.019521 -1.019521 -1 -1 -1 -0.311758 -0.311758 -0.311758 0 0 0 0.001043 0.001043 0.001043 0.001043
  line L145 (-4.8441, -21.5882) -> (-4.0922, -21.7445)
  line L146 (-5.5908, -21.4082) -> (-4.8441, -21.5882)
  spline S73 degree 3 poles (-5.9276, -17.8387) (-5.9279, -17.8398) (-5.9281, -17.8409) (-5.9284, -17.842) (-6.074, -18.391) (-6.0491, -18.9641) (-5.9878, -19.539) (-5.9242, -20.1352) (-5.794, -20.7379) (-5.6115, -21.3398) (-5.6046, -21.3626) (-5.5977, -21.3854) (-5.5908, -21.4082) knots -0.001043 -0.001043 -0.001043 -0.001043 0 0 0 0.490911 0.490911 0.490911 1 1 1 1.019521 1.019521 1.019521 1.019521
  line L147 (-5.679, -17.0738) -> (-5.9276, -17.8387)
  arc A112 (-5.679, -17.0738) -> (-5.9099, -16.6046) centre (-6.0357, -16.9579) ccw
  arc A113 (-7.085, -16.1383) -> (-5.9099, -16.6046) centre (0, 0) ccw
  arc A114 (-7.085, -16.1383) -> (-7.5748, -16.3214) centre (-7.2357, -16.4816) ccw
  line L148 (-7.9184, -17.0485) -> (-7.5748, -16.3214)
  spline S74 degree 3 poles (-10.6113, -19.4157) (-10.5906, -19.4038) (-10.5699, -19.392) (-10.5493, -19.3801) (-9.8117, -18.9571) (-9.1396, -18.4691) (-8.5817, -17.8992) (-8.329, -17.641) (-8.0918, -17.3687) (-7.92, -17.0516) (-7.9195, -17.0506) (-7.9189, -17.0496) (-7.9184, -17.0485) knots -1.019521 -1.019521 -1.019521 -1.019521 -1 -1 -1 -0.311758 -0.311758 -0.311758 0 0 0 0.001043 0.001043 0.001043 0.001043
  line L149 (-11.2782, -19.0347) -> (-10.6113, -19.4157)
  line L150 (-11.9326, -18.6328) -> (-11.2782, -19.0347)
  spline S75 degree 3 poles (-11.1499, -15.1339) (-11.1505, -15.1348) (-11.1511, -15.1358) (-11.1518, -15.1367) (-11.4599, -15.6139) (-11.6132, -16.1667) (-11.7326, -16.7324) (-11.8564, -17.319) (-11.9188, -17.9325) (-11.9312, -18.5613) (-11.9317, -18.5851) (-11.9322, -18.609) (-11.9326, -18.6328) knots -0.001043 -0.001043 -0.001043 -0.001043 0 0 0 0.490911 0.490911 0.490911 1 1 1 1.019521 1.019521 1.019521 1.019521
  line L151 (-10.6772, -14.4832) -> (-11.1499, -15.1339)
  arc A115 (-10.6772, -14.4832) -> (-10.7518, -13.9657) centre (-10.9806, -14.2628) ccw
  arc A116 (-11.7252, -13.159) -> (-10.7518, -13.9657) centre (0, 0) ccw
  arc A117 (-11.7252, -13.159) -> (-12.2476, -13.1819) centre (-11.9747, -13.439) ccw
  line L152 (-12.7991, -13.7672) -> (-12.2476, -13.1819)
  spline S76 degree 3 poles (-16.0918, -15.1864) (-16.0684, -15.1815) (-16.0451, -15.1766) (-16.0217, -15.1717) (-15.1896, -14.9972) (-14.3995, -14.7409) (-13.6928, -14.3712) (-13.3727, -14.2038) (-13.063, -14.0181) (-12.8016, -13.7696) (-12.8008, -13.7688) (-12.7999, -13.768) (-12.7991, -13.7672) knots -1.019521 -1.019521 -1.019521 -1.019521 -1 -1 -1 -0.311758 -0.311758 -0.311758 0 0 0 0.001043 0.001043 0.001043 0.001043
  line L153 (-16.6082, -14.6179) -> (-16.0918, -15.1864)
  line L154 (-17.1065, -14.0335) -> (-16.6082, -14.6179)
  spline S77 degree 3 poles (-15.2808, -10.9476) (-15.2817, -10.9484) (-15.2826, -10.9491) (-15.2835, -10.9498) (-15.7239, -11.3084) (-16.0406, -11.7867) (-16.3289, -12.2879) (-16.6279, -12.8075) (-16.8769, -13.3717) (-17.083, -13.9659) (-17.0908, -13.9884) (-17.0987, -14.0109) (-17.1065, -14.0335) knots -0.001043 -0.001043 -0.001043 -0.001043 0 0 0 0.490911 0.490911 0.490911 1 1 1 1.019521 1.019521 1.019521 1.019521
  line L155 (-14.6302, -10.4749) -> (-15.2808, -10.9476)
  arc A118 (-14.6302, -10.4749) -> (-14.5412, -9.9596) centre (-14.8506, -10.1715) ccw
  arc A119 (-15.2177, -8.8917) -> (-14.5412, -9.9596) centre (0, 0) ccw
  arc A120 (-15.2177, -8.8917) -> (-15.7216, -8.752) centre (-15.5415, -9.0809) ccw
  line L156 (-16.427, -9.1383) -> (-15.7216, -8.752)
  spline S78 degree 3 poles (-19.997, -9.4705) (-19.9733, -9.473) (-19.9496, -9.4756) (-19.9259, -9.4781) (-19.0805, -9.5694) (-18.2499, -9.5697) (-17.4636, -9.4366) (-17.1074, -9.3763) (-16.7555, -9.2954) (-16.4301, -9.1397) (-16.429, -9.1392) (-16.428, -9.1388) (-16.427, -9.1383) knots -1.019521 -1.019521 -1.019521 -1.019521 -1 -1 -1 -0.311758 -0.311758 -0.311758 0 0 0 0.001043 0.001043 0.001043 0.001043
  line L157 (-20.3125, -8.7702) -> (-19.997, -9.4705)
  line L158 (-20.6058, -8.0604) -> (-20.3125, -8.7702)
  spline S79 degree 3 poles (-17.9159, -5.6898) (-17.917, -5.6902) (-17.918, -5.6906) (-17.9191, -5.691) (-18.4488, -5.8959) (-18.8978, -6.253) (-19.3269, -6.6405) (-19.7718, -7.0424) (-20.183, -7.502) (-20.5626, -8.0034) (-20.577, -8.0224) (-20.5914, -8.0414) (-20.6058, -8.0604) knots -0.001043 -0.001043 -0.001043 -0.001043 0 0 0 0.490911 0.490911 0.490911 1 1 1 1.019521 1.019521 1.019521 1.019521
  line L159 (-17.151, -5.4413) -> (-17.9159, -5.6898)
  circle A121 centre (0, 0) radius 2.325
  dimension "d23" = 0.125
  dimension "d24" = -0.125
hidden bodies 5
equation "modulus = 2 mm"
equation "numteeth = 20"
equation "pressureangle = 20 deg"
equation "pitchdiameter = modulus * numteeth"
equation "basediameter = pitchdiameter * cos(pressureangle)"
equation "addendum = 1 * modulus"
equation "dedendum = 1.25 * modulus"
equation "addendumdiameter = pitchdiameter + 2 * addendum"
equation "dedendumdiameter = pitchdiameter - 2 * dedendum"
equation "d10 = pitchdiameter"
equation "d11 = basediameter"
equation "d12 = dedendumdiameter"
equation "d13 = addendumdiameter"
equation "d14 = ( ( 360 / numteeth / 2 / 2 ) * 1 deg ) + 0.853 deg"
equation "d20 = numteeth"
equation "kerf = 0.25 mm"
equation "d23 = kerf / 2"
equation "d24 = -kerf / 2"

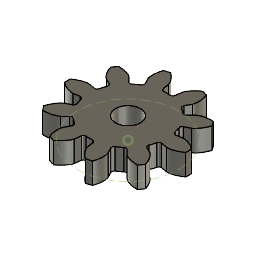
design "Spur Gear 2"
part number: 2026-02-17-13-56-46-487
Autodesk Fusion 360 part; units mm, degrees
sketch "Base Circle" plane through (0, 0, 0) normal (0, 0, 1) x (1, 0, 0)
  circle A0 centre (0, 0) radius 7.686
  circle A1 centre (0, 0) radius 2.45
extrude "Extrude1" add sketch "Base Circle" along normal blind 4.2
sketch "Gear Tooth" plane through (0, 0, 0) normal (0, 0, 1) x (1, 0, 0)
  spline S0 degree 5 poles (9.2583, -1.6082) (9.2659, -1.6095) (9.2813, -1.6119) (9.3043, -1.6147) (9.3352, -1.6169) (9.374, -1.6176) (9.413, -1.6169) (9.4522, -1.6152) (9.4913, -1.6131) (9.5306, -1.6106) (9.5699, -1.6078) (9.6092, -1.6044) (9.6485, -1.6005) (9.688, -1.5957) (9.7275, -1.5903) (9.767, -1.5842) (9.8065, -1.5774) (9.8461, -1.5702) (9.8857, -1.5626) (9.9253, -1.5546) (9.9649, -1.5461) (10.0045, -1.5372) (10.0441, -1.5278) (10.0838, -1.5179) (10.1234, -1.5076) (10.163, -1.4969) (10.2027, -1.4857) (10.2423, -1.4741) (10.2819, -1.4621) (10.3215, -1.4497) (10.3611, -1.4369) (10.4006, -1.4237) (10.4402, -1.4102) (10.4797, -1.3962) (10.5192, -1.3819) (10.5587, -1.3672) (10.5982, -1.3521) (10.6376, -1.3367) (10.677, -1.3209) (10.7163, -1.3047) (10.7557, -1.2882) (10.795, -1.2713) (10.8342, -1.2541) (10.8734, -1.2366) (10.9126, -1.2187) (10.9517, -1.2004) (10.9908, -1.1818) (11.0298, -1.1629) (11.0688, -1.1437) (11.1078, -1.1241) (11.1466, -1.1042) (11.1855, -1.084) (11.2242, -1.0634) (11.2629, -1.0425) (11.3016, -1.0213) (11.3402, -0.9998) (11.3787, -0.978) (11.4172, -0.9559) (11.4556, -0.9334) (11.4939, -0.9107) (11.5322, -0.8876) (11.5704, -0.8642) (11.6085, -0.8406) (11.6466, -0.8166) (11.6846, -0.7923) (11.7225, -0.7677) (11.7603, -0.7429) (11.7981, -0.7177) (11.8358, -0.6923) (11.8733, -0.6665) (11.9109, -0.6405) (11.9408, -0.6194) (11.9632, -0.6035) (11.9781, -0.5928) (11.9856, -0.5875) knots 0 0 0 0 0 0 0.01428571 0.02857143 0.04285714 0.05714286 0.07142857 0.08571429 0.1 0.11428571 0.12857143 0.14285714 0.15714286 0.17142857 0.18571429 0.2 0.21428571 0.22857143 0.24285714 0.25714286 0.27142857 0.28571429 0.3 0.31428571 0.32857143 0.34285714 0.35714286 0.37142857 0.38571429 0.4 0.41428571 0.42857143 0.44285714 0.45714286 0.47142857 0.48571429 0.5 0.51428571 0.52857143 0.54285714 0.55714286 0.57142857 0.58571429 0.6 0.61428571 0.62857143 0.64285714 0.65714286 0.67142857 0.68571429 0.7 0.71428571 0.72857143 0.74285714 0.75714286 0.77142857 0.78571429 0.8 0.81428571 0.82857143 0.84285714 0.85714286 0.87142857 0.88571429 0.9 0.91428571 0.92857143 0.94285714 0.95714286 0.97142857 0.98571429 1 1 1 1 1 1
  spline S1 degree 5 poles (9.2583, 1.6082) (9.2659, 1.6095) (9.2813, 1.6119) (9.3043, 1.6147) (9.3352, 1.6169) (9.374, 1.6176) (9.413, 1.6169) (9.4522, 1.6152) (9.4913, 1.6131) (9.5306, 1.6106) (9.5699, 1.6078) (9.6092, 1.6044) (9.6485, 1.6005) (9.688, 1.5957) (9.7275, 1.5903) (9.767, 1.5842) (9.8065, 1.5774) (9.8461, 1.5702) (9.8857, 1.5626) (9.9253, 1.5546) (9.9649, 1.5461) (10.0045, 1.5372) (10.0441, 1.5278) (10.0838, 1.5179) (10.1234, 1.5076) (10.163, 1.4969) (10.2027, 1.4857) (10.2423, 1.4741) (10.2819, 1.4621) (10.3215, 1.4497) (10.3611, 1.4369) (10.4006, 1.4237) (10.4402, 1.4102) (10.4797, 1.3962) (10.5192, 1.3819) (10.5587, 1.3672) (10.5982, 1.3521) (10.6376, 1.3367) (10.677, 1.3209) (10.7163, 1.3047) (10.7557, 1.2882) (10.795, 1.2713) (10.8342, 1.2541) (10.8734, 1.2366) (10.9126, 1.2187) (10.9517, 1.2004) (10.9908, 1.1818) (11.0298, 1.1629) (11.0688, 1.1437) (11.1078, 1.1241) (11.1466, 1.1042) (11.1855, 1.084) (11.2242, 1.0634) (11.2629, 1.0425) (11.3016, 1.0213) (11.3402, 0.9998) (11.3787, 0.978) (11.4172, 0.9559) (11.4556, 0.9334) (11.4939, 0.9107) (11.5322, 0.8876) (11.5704, 0.8642) (11.6085, 0.8406) (11.6466, 0.8166) (11.6846, 0.7923) (11.7225, 0.7677) (11.7603, 0.7429) (11.7981, 0.7177) (11.8358, 0.6923) (11.8733, 0.6665) (11.9109, 0.6405) (11.9408, 0.6194) (11.9632, 0.6035) (11.9781, 0.5928) (11.9856, 0.5875) knots 0 0 0 0 0 0 0.01428571 0.02857143 0.04285714 0.05714286 0.07142857 0.08571429 0.1 0.11428571 0.12857143 0.14285714 0.15714286 0.17142857 0.18571429 0.2 0.21428571 0.22857143 0.24285714 0.25714286 0.27142857 0.28571429 0.3 0.31428571 0.32857143 0.34285714 0.35714286 0.37142857 0.38571429 0.4 0.41428571 0.42857143 0.44285714 0.45714286 0.47142857 0.48571429 0.5 0.51428571 0.52857143 0.54285714 0.55714286 0.57142857 0.58571429 0.6 0.61428571 0.62857143 0.64285714 0.65714286 0.67142857 0.68571429 0.7 0.71428571 0.72857143 0.74285714 0.75714286 0.77142857 0.78571429 0.8 0.81428571 0.82857143 0.84285714 0.85714286 0.87142857 0.88571429 0.9 0.91428571 0.92857143 0.94285714 0.95714286 0.97142857 0.98571429 1 1 1 1 1 1
  arc A0 (11.9856, -0.5875) -> (11.9856, 0.5875) centre (0, 0) ccw
  line L0 (7.5628, -1.3137) -> (9.2583, -1.6082)
  line L1 (7.5628, 1.3137) -> (9.2583, 1.6082)
  line L2 (7.5628, -1.3137) -> (7.5628, 1.3137)
  point P0 (9.4457, -1.6154)
  point P1 (9.6366, -1.6016)
  point P2 (9.8296, -1.5732)
  point P3 (10.0242, -1.5325)
  point P4 (10.2199, -1.4806)
  point P5 (10.4164, -1.4183)
  point P6 (10.6134, -1.3461)
  point P7 (10.8107, -1.2644)
  point P8 (11.008, -1.1735)
  point P9 (11.205, -1.0736)
  point P10 (11.4014, -0.9649)
  point P11 (11.5972, -0.8476)
  point P12 (11.792, -0.7217)
  point P13 (9.4457, 1.6154)
  point P14 (9.6366, 1.6016)
  point P15 (9.8296, 1.5732)
  point P16 (10.0242, 1.5325)
  point P17 (10.2199, 1.4806)
  point P18 (10.4164, 1.4183)
  point P19 (10.6134, 1.3461)
  point P20 (10.8107, 1.2644)
  point P21 (11.008, 1.1735)
  point P22 (11.205, 1.0736)
  point P23 (11.4014, 0.9649)
  point P24 (11.5972, 0.8476)
  point P25 (11.792, 0.7217)
extrude "Extrude2" add sketch "Gear Tooth" along normal blind 4.2
fillet "Fillet1" radius 0.5 2 edges at (7.5726, -1.3154, 2.1) (7.5726, 1.3154, 2.1)
pattern_circular "C-Pattern1" count 10 over 360 about axis through (0, 0, 0) along (0, 0, 1) of "Extrude2", "Fillet1"
sketch "Diametrial Pitch Circle" plane through (0, 0, 0) normal (0, 0, 1) x (1, 0, 0)
  circle A0 centre (0, 0) radius 10 construction
named bodies: "Spur Gear (10 teeth)"
